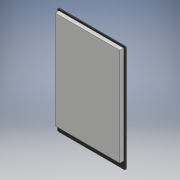
# Autodesk Inventor part: LCD+Cover
Saved by Autodesk Inventor 2017 (Build 210142000, 142)
## iProperties
Created: 2018-08-02
Part Number: LCD+Cover
Material: Generic
Document SubType Name: Modeling
Designer: intelsath
Density: 1 g/cm^3
Appearance: Default
Author: intelsath
Autodesk Inventor part; units mm, degrees
ref_plane "YZ Plane" through (0, 0, 0) normal (1, 0, 0) x (0, 1, 0)
ref_plane "XZ Plane" through (0, 0, 0) normal (0, 1, 0) x (-1, 0, 0)
ref_plane "XY Plane" through (0, 0, 0) normal (0, 0, 1) x (1, 0, 0)
sketch "Sketch1" plane through (0, 0, 0) normal (0, 1, 0) x (-1, 0, 0)
  line L0 (0, 0) -> (-54.66, 0)
  line L1 (-54.66, 0) -> (-54.66, -82.94)
  line L2 (-54.66, -82.94) -> (0, -82.94)
  line L3 (0, -82.94) -> (0, 0)
  dimension "d0" = 54.66
  dimension "d1" = 82.94
  constraints: 8 end point, 2 parallel, 1 horizontal, 1 perpendicular
  measures "d0" distance of L0.start L0.end
  measures "d1" distance of L0.end L1.end
extrude "Extrusion1" add sketch "Sketch1" along normal blind 2.3
sketch "Sketch2" plane through (0, 2.3, 0) normal (0, 1, 0) x (1, 0, 0)
  point P0 (0, 0)
sketch "Sketch3" plane through (0, 2.3, 0) normal (0, 1, 0) x (1, 0, 0)
  line L0 (2.85, 7.15) -> (51.81, 7.15)
  line L1 (51.81, 7.15) -> (51.81, 80.59)
  line L2 (51.81, 80.59) -> (2.85, 80.59)
  line L3 (2.85, 80.59) -> (2.85, 7.15)
  line L4 (54.66, 82.94) -> (0, 82.94) projected
  line L5 (0, 82.94) -> (0, 0) projected
  line L6 (0, 0) -> (54.66, 0)
  line L7 (54.66, 0) -> (54.66, 82.94)
  line L8 (54.66, 82.94) -> (0, 82.94)
  line L9 (0, 82.94) -> (0, 0)
  dimension "d4" = 73.44
  dimension "d5" = 48.96
  dimension "d6" = 2.35
  dimension "d7" = 2.85
  constraints: 16 end point, 4 parallel, 2 horizontal, 2 perpendicular
  measures "d4" distance of L2.end L0.start
  measures "d5" distance of L1.end L2.end
  measures "d6" distance between parallel lines of L4 L2
  measures "d7" distance between parallel lines of L5 L3
extrude "Extrusion2" add sketch "Sketch3" along normal blind 1
sketch "Sketch4" plane through (0, 3.3, 0) normal (0, 1, 0) x (1, 0, 0)
  line L0 (-1.52, -1.5) -> (56.18, -1.5)
  line L1 (56.18, -1.5) -> (56.18, 89.1)
  line L2 (56.18, 89.1) -> (-1.52, 89.1)
  line L3 (-1.52, 89.1) -> (-1.52, -1.5)
  line L4 (0, 0) -> (54.66, 0) projected
  line L5 (54.66, 82.94) -> (0, 82.94) projected
  line L6 (2.85, 7.15) -> (51.81, 7.15) projected
  line L7 (51.81, 80.59) -> (2.85, 80.59) projected
  line L8 (51.81, 7.15) -> (2.85, 7.15)
  line L9 (2.85, 7.15) -> (2.85, 80.59)
  line L10 (2.85, 80.59) -> (51.81, 80.59)
  line L11 (51.81, 80.59) -> (51.81, 7.15)
  point P0 (27.33, 82.94)
  point P1 (27.33, 89.1)
  dimension "d10" = 90.6
  dimension "d11" = 57.7
  dimension "d12" = 1.5
  constraints: 16 end point, 4 parallel, 2 horizontal, 2 midpoint, 2 perpendicular, 1 vertical alignment
  measures "d10" distance of L2.end L0.start
  measures "d11" distance of L1.end L2.end
  measures "d12" distance between parallel lines of L0 L4
extrude "Extrusion3" add sketch "Sketch4" along normal blind 0.7
fillet "Fillet1" radius 1 4 edges at (-1.52, 3.65, 1.5) (56.18, 3.65, 1.5) (56.18, 3.65, -89.1) (-1.52, 3.65, -89.1)
sketch "Sketch5" plane through (0, 2.3, 0) normal (0, 1, 0) x (1, 0, 0)
  line L0 (51.81, 7.15) -> (2.85, 7.15) projected
  line L1 (2.85, 80.59) -> (51.81, 80.59) projected
  line L2 (2.85, 7.15) -> (51.81, 7.15)
  line L3 (51.81, 7.15) -> (51.81, 80.59)
  line L4 (51.81, 80.59) -> (2.85, 80.59)
  line L5 (2.85, 80.59) -> (2.85, 7.15)
  point P0 (0, 0)
  constraints: 8 end point, 2 parallel, 1 horizontal, 1 perpendicular
extrude "Extrusion4" add sketch "Sketch5" along normal blind 1.6999
sketch "Sketch6" plane through (0, 4, 0) normal (0, 1, 0) x (1, 0, 0)
  line L0 (2.9162, 87.2914) -> (51.6645, 87.2914) construction
  line L1 (51.6645, 87.2914) -> (51.6645, 82.2368) construction
  line L2 (51.6645, 82.2368) -> (2.9162, 82.2368) construction
  line L3 (2.9162, 82.2368) -> (2.9162, 87.2914) construction
  constraints: 2 other
body "Solid1"
